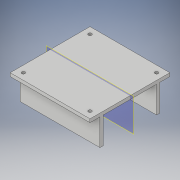
# Autodesk Inventor part: Right Angle Frame Mount
Saved by Autodesk Inventor 2019 (Build 230136000, 136)
## iProperties
Created: 2018-10-28
Part Number: Right Angle Frame Mount
Material: Generic
Document SubType Name: Modeling
Designer: Swapnil
Density: 1 g/cm^3
Appearance: Default
Mass: 30.6252 g
Surface Area: 207.085 cm^2
Volume: 30.6252 cm^3
Author: Swapnil
Autodesk Inventor part; units mm, degrees
ref_plane "YZ Plane" through (0, 0, 0) normal (1, 0, 0) x (0, 1, 0)
ref_plane "XZ Plane" through (0, 0, 0) normal (0, 1, 0) x (-1, 0, 0)
sketch "Sketch1" plane through (0, 0, 0) normal (0, 1, 0) x (-1, 0, 0)
  line L0 (0, 0) -> (4.388, 0) construction
  line L1 (4.1982, 0) -> (0, 0) construction
  line L2 (0, 0) -> (0, -4.5146) construction
  line L3 (38.1, 38.1) -> (-38.1, 38.1)
  line L4 (-38.1, 38.1) -> (-38.1, -38.1)
  line L5 (-38.1, -38.1) -> (38.1, -38.1)
  line L6 (38.1, -38.1) -> (38.1, 38.1)
  dimension "d0" = 76.2
  dimension "d1" = 76.2
  constraints: 14 end point, 3 horizontal, 2 parallel, 1 perpendicular, 1 point on line, 1 vertical, 2 other
  measures "d0" distance of L4.end L5.end
  measures "d1" distance of L5.end L3.start
extrude "Extrusion1" add sketch "Sketch1" along normal blind 3.175
ref_plane "Work Plane1" through (0, 0, 25.4) normal (0, 0, 1) x (1, 0, 0)
sketch "Sketch2" plane through (0, 0, 0) normal (0, -1, 0) x (1, 0, 0)
  line L0 (38.1, 38.1) -> (38.1, -38.1) projected
  line L1 (-38.1, -38.1) -> (-38.1, 38.1) projected
  line L2 (38.1, 25.3924) -> (-38.1, 25.3924)
  line L3 (-38.1, 25.3924) -> (-38.1, 28.5674)
  line L4 (-38.1, 28.5674) -> (38.1, 28.5674)
  line L5 (38.1, 28.5674) -> (38.1, 25.3924)
  point P0 (0, 0)
  dimension "d5" = 3.175
  constraints: 8 end point, 2 parallel, 2 point on line, 1 horizontal, 1 perpendicular
  measures "d5" distance between parallel lines of L2 L4
extrude "Extrusion2" add sketch "Sketch2" along normal blind 25.4
mirror "Mirror1" about plane through (0, 0, 0) normal (0, 0, 1) of "Extrusion2"
sketch "Sketch3" plane through (0, 3.175, 0) normal (0, 1, 0) x (1, 0, 0)
  line L0 (-38.1, 38.1) -> (-38.1, -38.1) projected
  line L1 (-38.1, -38.1) -> (38.1, -38.1) projected
  point P0 (0, 0)
  point P1 (-31.75, -31.75)
  dimension "d8" = 6.35
  dimension "d9" = 6.35
  measures "d8" distance from line of L0 point (-31.75, -31.75)
  measures "d9" distance from line of L1 point (-31.75, -31.75)
hole "Hole1" at (-31.75, 3.175, 31.75) direction (0, -1, 0) diameter 3.175 end through all
mirror "Mirror2" about plane through (0, 0, 0) normal (1, 0, 0) of "Hole1"
mirror "Mirror3" about plane through (0, 0, 0) normal (0, 0, 1) of "Hole1", "Mirror2"
ref_plane "Work Plane2" through (0, 0, 0) normal (0, 0, 1) x (1, 0, 0)
body "Solid1"
